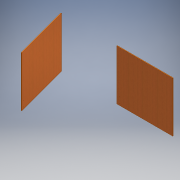
# Autodesk Inventor part: puerta
Saved by Autodesk Inventor 2016 (Build 200138000, 138)
## iProperties
Created: 2015-11-25
Part Number: puerta
Material: Generic
Document SubType Name: Modeling
Designer: Daniela
Density: 1 g/cm^3
Appearance: Glossy - Black
Author: Daniela
Autodesk Inventor part; units mm, degrees
ref_plane "YZ Plane" through (0, 0, 0) normal (1, 0, 0) x (0, 1, 0)
ref_plane "XZ Plane" through (0, 0, 0) normal (0, 1, 0) x (-1, 0, 0)
ref_plane "XY Plane" through (0, 0, 0) normal (0, 0, 1) x (1, 0, 0)
ref_plane "Plano de trabajo4" through (0, 0, 1220) normal (0, 0, 1) x (1, 0, 0)
sketch "Boceto8" plane through (0, 0, 1220) normal (0, 0, 1) x (1, 0, 0)
  line L0 (480, 0) -> (0, 0) projected
  line L1 (480, 0) -> (480, 10) projected
  line L2 (0, 10) -> (480, 10) projected
  line L3 (0, 0) -> (0, 10) projected
  line L4 (480, 10) -> (0, 10) projected
  line L5 (0, 10) -> (0, 300)
  line L6 (0, 300) -> (848.75, 300)
  line L7 (848.75, 300) -> (848.75, 310)
  line L8 (848.75, 310) -> (0, 310)
  line L9 (0, 310) -> (0, 300)
  point P0 (0, 0)
  dimension "d38" = 290
  dimension "d39" = 848.75
  dimension "d40" = 10
  constraints: 10 end point, 2 parallel, 1 horizontal, 1 perpendicular, 1 vertical
  measures "d38" distance of L2.start L5.end
  measures "d39" distance of L8.end L7.end
  measures "d40" distance of L7.end L6.end
extrude "Extrusión8" add sketch "Boceto8" along normal blind 730 contours L9 L8 L7 L6
sketch "Boceto9" plane through (0, 300, 1220) normal (0, -1, 0) x (1, 0, 0)
  line L0 (0, 0) -> (848.75, 0) construction
  line L1 (848.75, 0) -> (848.75, 730) construction
  line L2 (0, 730) -> (848.75, 730) construction
  line L3 (0, 0) -> (0, 730) construction
  line L4 (0, 80) -> (848.75, 80) construction
  line L5 (0, 0) -> (848.75, 0) construction
  line L6 (42.4375, 0) -> (42.4375, 730) construction
  line L7 (0, 730) -> (848.75, 730) construction
  circle A0 centre (42.4375, 30) radius 3
  circle A1 centre (42.4375, 130) radius 3
  point P0 (0, -1220)
  dimension "d43" = 42.4375
  dimension "d44" = 80
  dimension "d45" = 6
  dimension "d46" = 50
  constraints: 5 point on line, 4 end point, 2 centre point, 2 perpendicular, 1 symmetric about line, 1 other
  measures "d43" distance between parallel lines of L6 L3
  measures "d44" distance between parallel lines of L4 L0
  measures "d45" diameter of A0
  measures "d46" distance from line of L4 A0.centre
extrude "Extrusión9" cut sketch "Boceto9" against normal up to next
sketch "Boceto10" plane through (0, 0, 1950) normal (0, 0, 1) x (1, 0, 0)
  line L0 (848.75, 310) -> (0, 310) projected
  line L1 (0, 310) -> (-848.75, 310)
  line L2 (-848.75, 310) -> (-629.0773, -509.8295)
  line L3 (-629.0773, -509.8295) -> (-638.7366, -512.4177)
  line L4 (-638.7366, -512.4177) -> (-858.4093, 307.4118)
  line L5 (-858.4093, 307.4118) -> (-848.75, 310)
  point P0 (0, 0)
  dimension "d49" = 848.75
  dimension "d50" = 848.75
  dimension "angulo" = 75
  dimension "d52" = 10
  dimension "d53" = 848.75
  constraints: 10 end point, 2 perpendicular, 1 horizontal
  measures "d49" distance of L0.end L1.end
  measures "d50" distance of L1.end L2.end
  measures "angulo" angle of L2 L1
  measures "d52" distance of L2.end L3.end
  measures "d53" distance of L3.end L4.end
extrude "Extrusión10" add sketch "Boceto10" against normal blind 730
sketch "Boceto11" plane through (-629.0773, -509.8295, 1950) normal (0.9659258, 0.258819, 0) x (0, 0, -1)
  line L0 (0, 848.75) -> (0, 0) construction
  line L1 (0, 0) -> (730, 0) construction
  line L2 (730, 848.75) -> (730, 0) construction
  line L3 (0, 848.75) -> (730, 848.75) construction
  line L4 (0, 848.75) -> (0, 0) construction
  line L5 (0, 42.4375) -> (730, 42.4375) construction
  line L6 (0, 0) -> (730, 0) construction
  line L7 (650, 0) -> (650, 848.75) construction
  line L8 (0, 848.75) -> (730, 848.75) construction
  circle A0 centre (700, 42.4375) radius 3
  circle A1 centre (600, 42.4375) radius 3
  point P0 (1950, 329.6403)
  dimension "d56" = 42.4375
  dimension "d57" = 80
  dimension "d58" = 6
  dimension "d59" = 50
  constraints: 5 point on line, 4 end point, 2 centre point, 2 perpendicular, 1 symmetric about line, 1 other
  measures "d56" distance between parallel lines of L1 L5
  measures "d57" distance between parallel lines of L2 L7
  measures "d58" diameter of A0
  measures "d59" distance from line of L7 A0.centre
extrude "Extrusión11" cut sketch "Boceto11" against normal up to next
equation "\"d39\" = ancho_m"
equation "\"d40\" = espesor"
equation "\"d43\" = 0.05 * ancho_m"
equation "\"d49\" = ancho_m"
equation "\"d50\" = ancho_m"
equation "\"d52\" = espesor"
equation "\"d53\" = ancho_m"
equation "\"d54\" = h_sup"
equation "\"d56\" = 0.05 * ancho_m"
equation "\"d60\" = h_sup"
equation "\"ancho_m\" = 848.75"
equation "\"espesor\" = 10"
equation "\"h_sup\" = 730"
body "Solid1"
